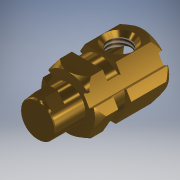
# Autodesk Inventor part: дз2 2
Saved by Autodesk Inventor 2019.3 (Build 233278000, 278)
## iProperties
Created: 2020-03-25
Part Number: дз2 2
Material: Латунь, мягкая, желтая
Document SubType Name: Modeling
Designer: Admin
Density: 8.47 g/cm^3
Appearance: Латунь — сатинированная
Mass: 16.7668 g
Surface Area: 21.9536 cm^2
Volume: 1.97955 cm^3
Author: Admin
Autodesk Inventor part; units mm, degrees
ref_plane "YZ Plane" through (0, 0, 0) normal (1, 0, 0) x (0, 1, 0)
ref_plane "XZ Plane" through (0, 0, 0) normal (0, 1, 0) x (-1, 0, 0)
ref_plane "XY Plane" through (0, 0, 0) normal (0, 0, 1) x (1, 0, 0)
sketch "Эскиз1" plane through (0, 0, 0) normal (0, 0, 1) x (1, 0, 0)
  line L0 (-4.0415, -7) -> (-8.0829, 0)
  line L1 (-8.0829, 0) -> (-4.0415, 7)
  line L2 (-4.0415, 7) -> (4.0415, 7)
  line L3 (4.0415, 7) -> (8.0829, 0)
  line L4 (8.0829, 0) -> (4.0415, -7)
  line L5 (4.0415, -7) -> (-4.0415, -7)
  point P0 (0, 0)
  point P1 (0, 0)
  dimension "d0" = 14
  constraints: 12 end point, 1 coincident, 1 horizontal alignment, 13 other
  measures "d0" distance between parallel lines of L5 L2
extrude "Выдавливание1" add sketch "Эскиз1" along normal blind 19.4
sketch "Эскиз2" plane through (0, 0, 19.4) normal (0, 0, 1) x (1, 0, 0)
  circle A0 centre (0, 0) radius 4.5
  dimension "d3" = 9
  constraints: 1 centre point, 1 coincident
  measures "d3" diameter of A0
extrude "Выдавливание2" add sketch "Эскиз2" along normal blind 8
sketch "Эскиз3" plane through (0, 0, 0) normal (0, 0, -1) x (-1, 0, 0)
  line L0 (-4.0415, -7) -> (4.0415, -7) projected
  point P0 (0, 0)
  point P1 (0, -0.675)
  dimension "d6" = 6.325
  measures "d6" distance from line of L0 point (0, -0.675)
hole "Отверстие1" at (0, -0.675, 0) direction (0, 0, 1) diameter 9.95 depth 18 tip angle 120
sketch "Эскиз5" plane through (0, 0, 0) normal (1, 0, 0) x (0, 1, 0)
  line L0 (-6.5, 14.4) -> (-6.5, 11)
  line L1 (-6.5, 11) -> (-15.5512, 11)
  line L2 (-15.5512, 11) -> (-15.5512, 14.4)
  line L3 (-15.5512, 14.4) -> (-6.5, 14.4)
  line L4 (0, 0) -> (0, 19.4) projected
  line L5 (-7, 19.4) -> (0, 19.4) projected
  line L6 (0, 0) -> (-7, 0) projected
  line L7 (0, -5.48) -> (0, 32.88) projected
  dimension "d21" = 6.5
  dimension "d22" = 5
  dimension "d23" = 11
  constraints: 8 end point, 2 horizontal, 2 vertical
  measures "d21" distance between parallel lines of L4 L0
  measures "d22" distance between parallel lines of L5 L3
  measures "d23" distance between parallel lines of L6 L1
revolve "Вращение1" cut sketch "Эскиз5" angle 360 about axis through (0, 0, -10) along (0, 0, 1)
sketch "Эскиз6" plane through (-4.0415, 7, 0) normal (0, 1, 0) x (1, 0, 0)
  line L0 (0, 0) -> (8.0829, 0) projected
  line L1 (4.0415, 5.48) -> (4.0415, -32.88) projected
  point P0 (4.0415, 0)
  point P1 (4.0415, 0)
  point P2 (4.0415, -6)
  dimension "d70" = 6
  constraints: 1 midpoint, 1 point on line
  measures "d70" distance of point (4.041, 0) point (4.041, -6)
ref_plane "РабПлоскость1" through (0, 0, 26.9) normal (0, 0, 1) x (1, 0, 0)
sketch "Эскиз7" plane through (0, 0, 26.9) normal (0, 0, 1) x (1, 0, 0)
  line L0 (-1.2214, 5.5) -> (1.2786, 5.5)
  circle A0 centre (0, 0) radius 4.5 projected
  line L1 (-1.2214, 5.5) -> (-3.4225, 2.9218)
  circle A1 centre (0, 0) radius 4.5 projected
  line L2 (1.2786, 5.5) -> (3.4597, 2.8775)
  arc A2 (-3.4225, 2.9218) -> (0, 4.5) centre (0, 0) ccw
  dimension "d32" = 2.5
  dimension "d33" = 5.5
  constraints: 6 end point, 5 point on circle, 2 tangent, 1 centre point, 1 concentric, 1 horizontal, 3 other
  measures "d32" distance of L0.start L0.end
  measures "d33" distance from line of point (0, 0) L0
extrude "Выдавливание5" add sketch "Эскиз7" against normal blind 3.4
chamfer "Фаска2" distance 0.2 angle 45 1 edges at (-4.5, 0, 27.4)
sketch "Эскиз8" plane through (0, 0, 0) normal (0, 1, 0) x (-1, 0, 0)
  line L0 (8.0829, 1.8756) -> (8.0829, 0)
  line L1 (8.0829, 0) -> (7, 0)
  line L2 (7, 0) -> (8.0829, 1.8756)
  line L3 (4.0415, 0) -> (8.0829, 0) projected
  line L4 (8.0829, 0) -> (8.0829, 11) projected
  line L5 (8.0829, 17.5244) -> (8.0829, 19.4)
  line L6 (8.0829, 19.4) -> (7, 19.4)
  line L7 (7, 19.4) -> (8.0829, 17.5244)
  line L8 (8.0829, 14.4) -> (8.0829, 19.4) projected
  line L9 (8.0829, 19.4) -> (4.0415, 19.4) projected
  line L10 (0, -5.48) -> (0, 32.88) projected
  point P0 (0, 0)
  dimension "d42" = 7
  dimension "d43" = 7
  dimension "d81" = 60
  constraints: 12 end point, 4 point on line, 1 collinear
  measures "d42" distance of point (0, 0) L1.end
  measures "d43" horizontal distance of point (0, 0) L6.end
  measures "d81" angle of L7 L6
revolve "Вращение2" cut sketch "Эскиз8" angle 360 about axis through (0, 0, -10) along (0, 0, 1)
sketch "Эскиз9" plane through (0, 0, 0) normal (0, 0, -1) x (-1, 0, 0)
  line L0 (-6.8122, 2.201) -> (-5.5131, 1.451)
  line L1 (-5.5131, 1.451) -> (-4.0131, 4.049)
  line L2 (-4.0131, 4.049) -> (-5.3122, 4.799)
  line L3 (-5.3122, 4.799) -> (-6.8122, 2.201)
  line L4 (-6.0622, 3.5) -> (-4.0415, 7) projected
  line L5 (-8.0829, 0) -> (-6.0622, 3.5) projected
  line L6 (-4.0415, 7) -> (-8.0829, 0)
  line L7 (-6.8122, 2.201) -> (-8.0829, 0)
  line L8 (-5.3122, 4.799) -> (-4.0415, 7)
  line L9 (0, -9.8) -> (0, 9.8) projected
  line L10 (6.8122, 2.201) -> (5.5131, 1.451)
  line L11 (5.5131, 1.451) -> (4.0131, 4.049)
  line L12 (4.0131, 4.049) -> (5.3122, 4.799)
  line L13 (5.3122, 4.799) -> (6.8122, 2.201)
  point P0 (0, 0)
  dimension "d64" = 3
  dimension "d65" = 1.5
  constraints: 22 end point, 4 symmetric about line, 3 perpendicular, 2 point on line, 1 collinear
  measures "d64" distance of L0.end L1.end
  measures "d65" distance of L1.end L2.end
extrude "Выдавливание7" cut sketch "Эскиз9" along normal through all both and the other way through all
hole "Отверстие2" at (0, 7, 6) direction (0, -1, 0) diameter 5.9175 end up to face face through (0, -0.675, 9) facing (0, 0, -1) round with radius 4.975 far side no thread size "M7x1" class "6H" standard "ISO Metric profile"
chamfer "Фаска5" distance 1 angle 45 1 edges at (0, 7, 3.0413)
